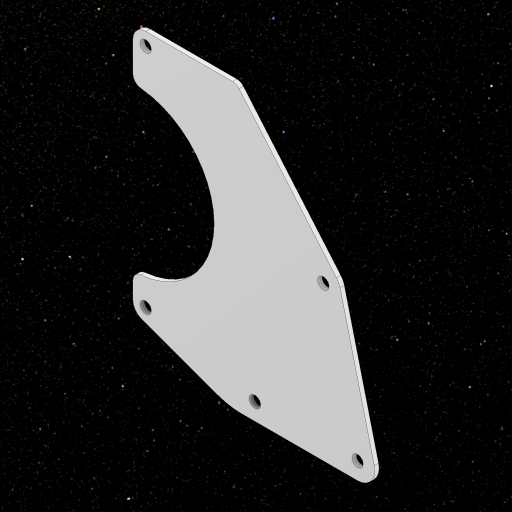
# Autodesk Inventor part: hang_gusset
Saved by Autodesk Inventor 2024 (Build 280153000, 153)
## iProperties
Created: 2024-02-16
Part Number: hang_gusset
Material: Acetal Resin, White
Document SubType Name: Modeling
Designer: Averey Ku
Density: 1.425 g/cm^3
Appearance: Smooth - White
Author: Averey Ku
Autodesk Inventor part; units mm, degrees
ref_plane "YZ Plane" through (0, 0, 0) normal (1, 0, 0) x (0, 1, 0)
ref_plane "XZ Plane" through (0, 0, 0) normal (0, 1, 0) x (-1, 0, 0)
ref_plane "XY Plane" through (0, 0, 0) normal (0, 0, 1) x (1, 0, 0)
sketch "main" plane through (0, 0, 0) normal (0, 0, 1) x (1, 0, 0)
  line L0 (57.2021, -70.0851) -> (14.0558, -70.0851)
  line L1 (5.3685, -68.5533) -> (-23.0916, -58.1947)
  line L2 (-26.2252, -53.7194) -> (-26.2252, -47.3776)
  arc A0 (-23.3526, -44.217) -> (-23.3526, 15.8337) centre (-26.2252, -14.1917) ccw
  line L3 (-26.2252, 18.9943) -> (-26.2252, 30.2583)
  line L4 (-21.4627, 35.0208) -> (10.7437, 35.0208)
  line L5 (13.1667, 33.8976) -> (49.3481, -8.8317)
  arc A1 (-21.4627, 35.0208) -> (-26.2252, 30.2583) centre (-21.4627, 30.2583) ccw
  circle A2 centre (-21.4627, 30.2583) radius 2.0955
  arc A3 (-26.2252, 18.9943) -> (-23.3526, 15.8337) centre (-23.0502, 18.9943) ccw
  arc A4 (-23.3526, -44.217) -> (-26.2252, -47.3776) centre (-23.0502, -47.3776) ccw
  arc A5 (-26.2252, -53.7194) -> (-23.0916, -58.1947) centre (-21.4627, -53.7194) ccw
  circle A6 centre (-21.4627, -53.7194) radius 2.0955
  arc A7 (13.1667, 33.8976) -> (10.7437, 35.0208) centre (10.7437, 31.8458) ccw
  circle A8 centre (57.2021, -63.7351) radius 2.0955
  arc A9 (50.6625, -11.395) -> (49.3481, -8.8317) centre (44.5021, -12.9351) ccw
  circle A10 centre (44.5021, -12.9351) radius 2.0955
  line L6 (50.6625, -11.395) -> (63.3625, -62.195)
  arc A11 (57.2021, -70.0851) -> (63.3625, -62.195) centre (57.2021, -63.7351) ccw
  circle A12 centre (19.1021, -63.7351) radius 2.0955
  arc A13 (5.3685, -68.5533) -> (14.0558, -70.0851) centre (14.0558, -44.6851) ccw
  point P0 (-12.3105, 3.8443)
  point P1 (9.5771, -70.0851)
  point P2 (-26.2252, -57.0542)
  point P3 (-26.2252, -44.3542)
  point P4 (-26.2252, 15.9708)
  point P5 (-26.2252, 35.0208)
  point P6 (20.6896, -70.0851)
  dimension "d14" = 38.1
  dimension "d15" = 160
  dimension "d16" = 12.7
  dimension "d17" = 19.05
  dimension "d18" = 4.7625
  dimension "d19" = 4.191
  dimension "d20" = 3.175
  dimension "d21" = 4.7625
  dimension "d22" = 4.191
  dimension "d23" = 4.191
  dimension "d24" = 4.191
  dimension "d25" = 4.191
  dimension "d26" = 25.4
  measures "d14" distance of point (9.577, -70.085) point (-26.225, -57.054)
  measures "d15" angle of L0 L1
  measures "d16" distance of point (-26.225, -57.054) point (-26.225, -44.354)
  measures "d17" distance of point (-26.225, 15.971) point (-26.225, 35.021)
  measures "d18" radius of A1
  measures "d19" diameter of A2
  measures "d20" radius of A3
  measures "d21" radius of A5
  measures "d22" diameter of A6
  measures "d23" diameter of A8
  measures "d24" diameter of A10
  measures "d25" diameter of A12
  measures "d26" radius of A13
sketch "Sketch1" plane through (0, 0, 0) normal (0, 0, 1) x (1, 0, 0)
  line L0 (78.6648, -100.3435) -> (35.5185, -100.3435)
  line L1 (26.8312, -98.8117) -> (-1.6289, -88.453)
  line L2 (-4.7625, -83.9778) -> (-4.7625, -77.636)
  arc A0 (-1.8899, -74.4754) -> (-1.8899, -14.4246) centre (-4.7625, -44.45) ccw
  line L3 (-4.7625, -11.264) -> (-4.7625, 0)
  line L4 (0, 4.7625) -> (32.2064, 4.7625)
  line L5 (34.6294, 3.6392) -> (70.8108, -39.09)
  arc A1 (0, 4.7625) -> (-4.7625, 0) centre (0, 0) ccw
  circle A2 centre (0, 0) radius 2.0955
  arc A3 (-4.7625, -11.264) -> (-1.8899, -14.4246) centre (-1.5875, -11.264) ccw
  arc A4 (-1.8899, -74.4754) -> (-4.7625, -77.636) centre (-1.5875, -77.636) ccw
  arc A5 (-4.7625, -83.9778) -> (-1.6289, -88.453) centre (0, -83.9778) ccw
  circle A6 centre (0, -83.9778) radius 2.0955
  arc A7 (34.6294, 3.6392) -> (32.2064, 4.7625) centre (32.2064, 1.5875) ccw
  circle A8 centre (78.6648, -93.9935) radius 2.0955
  arc A9 (72.1252, -41.6534) -> (70.8108, -39.09) centre (65.9648, -43.1935) ccw
  circle A10 centre (65.9648, -43.1935) radius 2.0955
  line L6 (72.1252, -41.6534) -> (84.8252, -92.4534)
  arc A11 (78.6648, -100.3435) -> (84.8252, -92.4534) centre (78.6648, -93.9935) ccw
  circle A12 centre (40.5648, -93.9935) radius 2.0955
  arc A13 (26.8312, -98.8117) -> (35.5185, -100.3435) centre (35.5185, -74.9435) ccw
  constraints: 1 other
extrude "Extrusion1" add sketch "Sketch1" along normal blind 1.5875
body "Solid1"
